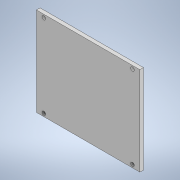
# Autodesk Inventor part: tapa
Saved by Autodesk Inventor 2020.3 (Build 243373000, 373)
## iProperties
Created: 2021-02-11
Part Number: tapa
Material: Generic
Document SubType Name: Modeling
Designer: Yu Jinyu
Density: 1 g/cm^3
Appearance: Default
Author: Yu Jinyu
Autodesk Inventor part; units mm, degrees
ref_plane "YZ Plane" through (0, 0, 0) normal (1, 0, 0) x (0, 1, 0)
ref_plane "XZ Plane" through (0, 0, 0) normal (0, 1, 0) x (-1, 0, 0)
ref_plane "XY Plane" through (0, 0, 0) normal (0, 0, 1) x (1, 0, 0)
sketch "Sketch1" plane through (0, 0, 0) normal (0, 0, 1) x (1, 0, 0)
  line L0 (-42.5, -36.45) -> (42.5, -36.45)
  line L1 (42.5, -36.45) -> (42.5, 36.45)
  line L2 (42.5, 36.45) -> (-42.5, 36.45)
  line L3 (-42.5, 36.45) -> (-42.5, -36.45)
  line L4 (-42.5, -36.45) -> (42.5, 36.45) construction
  line L5 (42.5, -36.45) -> (-42.5, 36.45) construction
  point P0 (0, 0)
  dimension "d0" = 85
  dimension "d1" = 72.9
  constraints: 12 end point, 2 midpoint, 2 parallel, 1 horizontal, 1 perpendicular
  measures "d0" distance of L2.end L1.end
  measures "d1" distance of L1.end L0.end
extrude "Extrusion1" add sketch "Sketch1" along normal blind 3
sketch "Sketch2" plane through (0, 0, 3) normal (0, 0, 1) x (1, 0, 0)
  circle A0 centre (-36.428, 33.95) radius 1.5
  circle A1 centre (36.428, 33.95) radius 1.5
  circle A2 centre (-36.428, -33.95) radius 1.5
  circle A3 centre (36.428, -33.95) radius 1.5
  line L0 (-42.5, 36.45) -> (-42.5, -36.45) projected
  line L1 (42.5, 36.45) -> (-42.5, 36.45) projected
  line L2 (42.5, -36.45) -> (42.5, 36.45) projected
  line L3 (-42.5, -36.45) -> (42.5, -36.45) projected
  point P0 (0, 0)
  dimension "d4" = 3
  dimension "d5" = 3
  dimension "d6" = 3
  dimension "d7" = 6.072
  dimension "d8" = 2.5
  dimension "d9" = 2.5
  dimension "d10" = 6.072
  dimension "d11" = 2.5
  dimension "d12" = 6.072
  dimension "d13" = 6.072
  dimension "d14" = 2.5
  constraints: 4 centre point
  measures "d4" diameter of A0
  measures "d5" diameter of A1
  measures "d6" diameter of A2
  measures "d7" distance from line of L0 A0.centre
  measures "d8" distance from line of L1 A0.centre
  measures "d9" distance from line of A1.centre L1
  measures "d10" distance from line of L2 A1.centre
  measures "d11" distance from line of L3 A2.centre
  measures "d12" distance from line of L0 A2.centre
  measures "d13" distance from line of L2 A3.centre
  measures "d14" distance from line of L3 A3.centre
extrude "Extrusion2" cut sketch "Sketch2" against normal blind 10 contours A0 | A1 | A2 | A3
body "Solid1"
